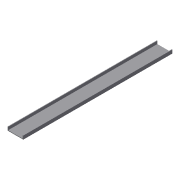
# Autodesk Inventor part: FrameSide
Saved by Autodesk Inventor 2015 (Build 190159000, 159)
## iProperties
Created: 2015-03-05
Part Number: FrameSide
Material: Generic
Document SubType Name: Modeling
Designer: Kyle
Density: 1 g/cm^3
Appearance: Default
Author: Kyle
Autodesk Inventor part; units mm, degrees
ref_plane "YZ Plane" through (0, 0, 0) normal (1, 0, 0) x (0, 1, 0)
ref_plane "XZ Plane" through (0, 0, 0) normal (0, 1, 0) x (-1, 0, 0)
ref_plane "XY Plane" through (0, 0, 0) normal (0, 0, 1) x (1, 0, 0)
sketch "Sketch1" plane through (0, 0, 0) normal (0, 0, 1) x (1, 0, 0)
  line L0 (0, 0) -> (0, 19.05)
  line L1 (0, 19.05) -> (3.175, 19.05)
  line L2 (3.175, 19.05) -> (3.175, 3.175)
  line L3 (3.175, 3.175) -> (82.55, 3.175)
  line L4 (0, 0) -> (85.725, 0)
  line L5 (0, 0) -> (85.725, 0) construction
  line L6 (85.725, 0) -> (85.725, 19.05)
  line L7 (82.55, 3.175) -> (82.55, 19.05)
  line L8 (82.55, 19.05) -> (85.725, 19.05)
  dimension "d7" = 19.05
  dimension "d8" = 3.175
  dimension "d9" = 15.875
  dimension "d10" = 79.375
  dimension "d11" = 90
  dimension "d12" = 85.725
  dimension "d13" = 0
  dimension "d14" = 19.05
  constraints: 18 end point, 5 perpendicular, 2 horizontal, 2 vertical, 1 collinear
  measures "d7" distance of L0.start L0.end
  measures "d8" distance of L0.end L1.end
  measures "d9" distance of L1.end L2.end
  measures "d10" distance of L2.end L3.end
  measures "d11" angle of L3 L2
  measures "d12" distance of L0.start L4.end
  measures "d13" distance between parallel lines of L4 L5
  measures "d14" distance of L4.end L6.end
extrude "Extrusion1" add sketch "Sketch1" along normal blind 812.8
body "Solid1"
